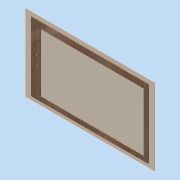
# Autodesk Inventor part: Part3
Saved by Autodesk Inventor 2017 (Build 210142000, 142)
## iProperties
Created: 2018-10-05
Part Number: Part3
Material: Wood (Birch)
Document SubType Name: Modeling
Designer: mailb
Density: 0.55 g/cm^3
Appearance: Birch - Natural Polished
Author: mailb
Autodesk Inventor part; units mm, degrees
ref_plane "YZ Plane" through (0, 0, 0) normal (1, 0, 0) x (0, 1, 0)
ref_plane "XZ Plane" through (0, 0, 0) normal (0, 1, 0) x (-1, 0, 0)
ref_plane "XY Plane" through (0, 0, 0) normal (0, 0, 1) x (1, 0, 0)
ref_plane "Work Plane1" through (0, 0, 0) normal (0, 0, 1) x (1, 0, 0)
sketch "Sketch1" plane through (0, 0, 0) normal (0, 0, 1) x (1, 0, 0)
  arc A0 (-261.52, -25.4) -> (-260.25, -24.13) centre (-261.52, -24.13) ccw projected
  line L0 (-261.52, -25.4) -> (-265.66, -25.4) projected
  arc A1 (-266.93, -24.13) -> (-265.66, -25.4) centre (-265.66, -24.13) ccw projected
  line L1 (-266.93, -24.13) -> (-266.93, -21.59) projected
  arc A2 (-265.66, -20.32) -> (-266.93, -21.59) centre (-265.66, -21.59) ccw projected
  line L2 (-265.66, -20.32) -> (-261.52, -20.32) projected
  arc A3 (-260.25, -21.59) -> (-261.52, -20.32) centre (-261.52, -21.59) ccw projected
  line L3 (-260.25, -21.59) -> (-260.25, -24.13) projected
  circle A4 centre (-264.3, 19.25) radius 3.6 projected
  arc A5 (291.2125, 168.0875) -> (288.0375, 171.2625) centre (288.0375, 168.0875) ccw projected
  line L4 (288.0375, 171.2625) -> (-288.0375, 171.2625) projected
  arc A6 (-288.0375, 171.2625) -> (-291.2125, 168.0875) centre (-288.0375, 168.0875) ccw projected
  line L5 (-291.2125, 168.0875) -> (-291.2125, -168.0875) projected
  arc A7 (-291.2125, -168.0875) -> (-288.0375, -171.2625) centre (-288.0375, -168.0875) ccw projected
  line L6 (-288.0375, -171.2625) -> (288.0375, -171.2625) projected
  arc A8 (288.0375, -171.2625) -> (291.2125, -168.0875) centre (288.0375, -168.0875) ccw projected
  line L7 (291.2125, -168.0875) -> (291.2125, 168.0875) projected
  point P0 (0, 0)
extrude "Extrusion1" add sketch "Sketch1" along normal blind 3.175
sketch "Sketch2" plane through (0, 0, 0) normal (0, 0, 1) x (1, 0, 0)
  arc A0 (267.27, -148.59) -> (268.54, -147.32) centre (267.27, -147.32) ccw projected
  line L0 (268.54, 140.97) -> (268.54, -147.32) projected
  line L1 (-244.54, 140.97) -> (268.54, 140.97) projected
  line L2 (-244.54, -147.32) -> (-244.54, 140.97) projected
  arc A1 (-244.54, -147.32) -> (-243.27, -148.59) centre (-243.27, -147.32) ccw projected
  line L3 (267.27, -148.59) -> (-243.27, -148.59) projected
  arc A2 (267.27, -148.59) -> (268.54, -147.32) centre (267.27, -147.32) ccw projected
  line L4 (268.54, 140.97) -> (268.54, -147.32) projected
  line L5 (-244.54, 140.97) -> (268.54, 140.97) projected
  line L6 (-244.54, -147.32) -> (-244.54, 140.97) projected
  arc A3 (-244.54, -147.32) -> (-243.27, -148.59) centre (-243.27, -147.32) ccw projected
  line L7 (267.27, -148.59) -> (-243.27, -148.59) projected
  point P0 (0, 0)
extrude "Extrusion2" cut sketch "Sketch2" along normal blind 3.175
body "Solid1"
